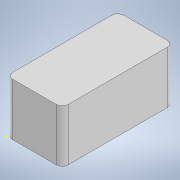
# Autodesk Inventor part: Capstone
Saved by Autodesk Inventor 2020 (Build 240168000, 168)
## iProperties
Created: 2020-02-01
Part Number: Capstone
Material: Generic
Document SubType Name: Modeling
Designer: xj82b
Density: 1 g/cm^3
Appearance: Default
Author: xj82b
Autodesk Inventor part; units mm, degrees
ref_plane "YZ Plane" through (0, 0, 0) normal (1, 0, 0) x (0, 1, 0)
ref_plane "XZ Plane" through (0, 0, 0) normal (0, 1, 0) x (-1, 0, 0)
ref_plane "XY Plane" through (0, 0, 0) normal (0, 0, 1) x (1, 0, 0)
sketch "Sketch1" plane through (0, 0, 0) normal (0, 1, 0) x (-1, 0, 0)
  line L0 (0, 0) -> (-88.9, 0)
  line L1 (-88.9, 0) -> (-88.9, -177.8)
  line L2 (-88.9, -177.8) -> (0, -177.8)
  line L3 (0, -177.8) -> (0, 0)
  dimension "d0" = 177.8
  dimension "d1" = 88.9
  constraints: 8 end point, 2 parallel, 1 horizontal, 1 perpendicular
  measures "d0" distance of L1.end L0.end
  measures "d1" distance of L1.end L2.end
extrude "Extrusion1" add sketch "Sketch1" along normal blind 83.82
sketch "Sketch2" plane through (0, 0, 0) normal (0, -1, 0) x (1, 0, 0)
  point P0 (0, 0)
sketch "Sketch3" plane through (0, 0, 0) normal (0, -1, 0) x (1, 0, 0)
  line L0 (88.9, 0) -> (88.9, -177.8) projected
  line L1 (0, 0) -> (88.9, 0) projected
  line L2 (0, -177.8) -> (0, 0) projected
  line L3 (88.9, -177.8) -> (0, -177.8) projected
  line L4 (76.0718, -164.9718) -> (76.0718, -12.8282)
  line L5 (76.0718, -12.8282) -> (12.8282, -12.8282)
  line L6 (12.8282, -12.8282) -> (12.8282, -164.9718)
  line L7 (12.8282, -164.9718) -> (76.0718, -164.9718)
  constraints: 8 end point, 3 other
extrude "Extrusion2" cut sketch "Sketch3" against normal blind 25.4 contours L7 L6 L5 L4
fillet "Fillet1" radius 10 4 edges at (88.9, 41.91, -177.8) (0, 41.91, -177.8) (88.9, 41.91, 0) (0, 41.91, 0)
body "Solid1"
